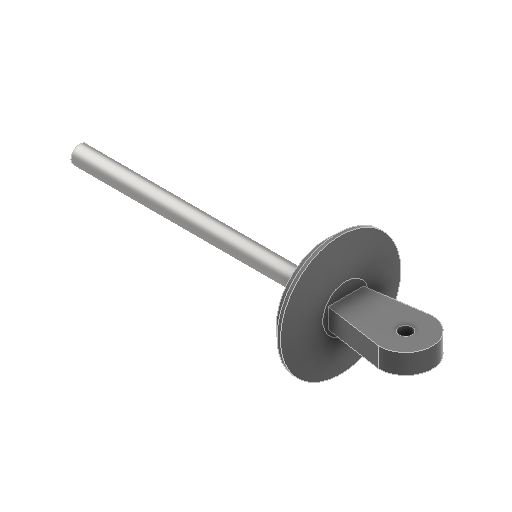
# Autodesk Inventor part: 100MMshockLower
Saved by Autodesk Inventor 2025 (Build 290162000, 162)
## iProperties
Created: 2024-10-22
Part Number: 100MMshockLower
Material: Generic
Document SubType Name: Modeling
Designer: derm
Density: 1 g/cm^3
Appearance: Smooth - Black
Author: derm
Autodesk Inventor part; units mm, degrees
ref_plane "YZ Plane" through (0, 0, 0) normal (1, 0, 0) x (0, 1, 0)
ref_plane "XZ Plane" through (0, 0, 0) normal (0, 1, 0) x (-1, 0, 0)
ref_plane "XY Plane" through (0, 0, 0) normal (0, 0, 1) x (1, 0, 0)
sketch "Sketch1" plane through (0, 0, 0) normal (0, 1, 0) x (-1, 0, 0)
  circle A0 centre (0, 0) radius 1.5
  circle A1 centre (0, 0) radius 6
  line L0 (13.4781, 0) -> (13.4781, -4)
  line L1 (13.4781, 0) -> (13.4781, 4)
  line L2 (13.4781, 4) -> (0, 6)
  line L3 (13.4781, -4) -> (0, -6)
  dimension "d0" = 3
  dimension "d1" = 12
  dimension "d2" = 4
  constraints: 8 end point, 2 centre point, 2 coincident, 2 point on circle, 2 vertical, 1 collinear
  measures "d0" diameter of A0
  measures "d1" diameter of A1
  measures "d2" distance of L0.start L1.end
extrude "Extrusion1" add sketch "Sketch1" along normal mid plane 4.5 contours L2 A1 L3 | L2 L1 L0 L3 A1
sketch "Sketch2" plane through (-13.4781, -2.25, -4) normal (-1, 0, 0) x (0, 0, 1)
  line L0 (2.5, 4.5) -> (2.5, 0) projected
  line L1 (8, 0) -> (0, 0) projected
  line L2 (8, 4.5) -> (8, 0) projected
  line L3 (0, 4.5) -> (8, 4.5) projected
  line L4 (0, 0) -> (0, 4.5) projected
  circle A0 centre (4, 2.25) radius 2
  dimension "d5" = 4
  constraints: 1 centre point
  measures "d5" diameter of A0
extrude "Extrusion2" add sketch "Sketch2" along normal blind 60 contours A0 L0 | L0 A0
fillet "Fillet1" [suppressed]
sketch "Sketch4" plane through (0, 0, 0) normal (0, 1, 0) x (-1, 0, 0)
  line L0 (13.4781, 4) -> (0, 6) projected
  arc A0 (0, 6) -> (0, -6) centre (0, 0) ccw projected
  line L1 (0, -6) -> (13.4781, -4) projected
  line L2 (13.4781, -4) -> (13.4781, 4) projected
  circle A1 centre (0, 0) radius 1.5 projected
  line L3 (13.4781, 4) -> (13.4781, -4) projected
  line L4 (13.4781, 0) -> (17.6846, 0)
  line L5 (17.6846, 0) -> (17.6846, 0.0214)
  line L6 (17.6846, -11.5062) -> (15.4451, -11.5062)
  line L7 (15.4451, -11.5062) -> (15.4451, -13.5813)
  line L8 (15.4451, -13.5813) -> (14.6622, -13.5813)
  line L9 (13.4781, -4) -> (13.4781, -5.198)
  line L10 (13.4781, -5.198) -> (14.6622, -13.5813)
  line L11 (17.6846, -11.5062) -> (17.6846, -10.8233)
  line L12 (17.6846, -10.8233) -> (15.4853, -10.8233)
  line L13 (15.4853, -10.8233) -> (15.0537, -7.0356)
  line L14 (15.0537, -7.0356) -> (15.0537, 0)
  dimension "d13" = 11.5062
  constraints: 22 end point, 4 vertical, 3 perpendicular, 2 point on line, 1 horizontal, 1 midpoint
  measures "d13" distance between parallel lines of L6 L4
revolve "Revolution1" add sketch "Sketch4" angle 360 about axis through (-13.4781, 0, 0) along (-1, 0, 0) contours L4 L14 L13 L12 L11 L6 L7 L8 L10 L9 L2
body "Solid1"
